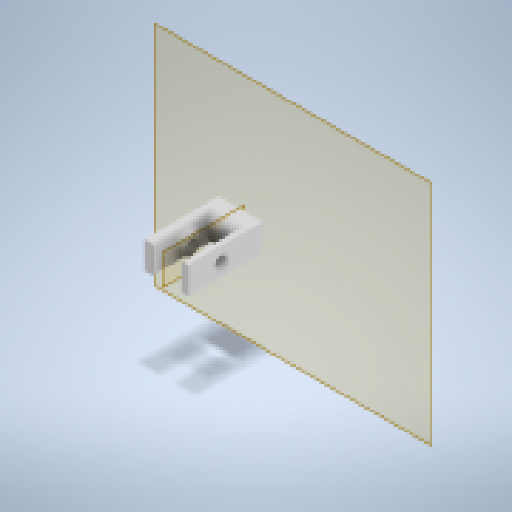
# Autodesk Inventor part: base-tensioner-head
Saved by Autodesk Inventor 2024 (Build 280153000, 153)
## iProperties
Created: 2024-03-29
Part Number: base-tensioner-head
Material: Generic
Document SubType Name: Modeling
Designer: MaartenGeorgesBuelen
Density: 1 g/cm^3
Appearance: Default
Author: MaartenGeorgesBuelen
## iProperties of the stored document base-tensioner-head_3DPrint.ipt
Created: 2024-04-17
Part Number: base-tensioner-head_3DPrint
Material: Generic
Document SubType Name: Modeling
Designer: MaartenGeorgesBuelen
Density: 1 g/cm^3
Appearance: Default
Author: MaartenGeorgesBuelen
Autodesk Inventor part; units mm, degrees
ref_plane "YZ Plane" through (0, 0, 0) normal (1, 0, 0) x (0, 1, 0)
ref_plane "XZ Plane" through (0, 0, 0) normal (0, 1, 0) x (-1, 0, 0)
ref_plane "XY Plane" through (0, 0, 0) normal (0, 0, 1) x (1, 0, 0)
ref_plane "Work Plane1" through (9.9569, 31.9885, -8.0612) normal (0, 0, 1) x (0.98136, 0.1921786, 0)
sketch "Sketch1" plane through (9.9569, 31.9885, -8.0612) normal (0, 0, 1) x (0.98136, 0.1921786, 0)
  line L0 (-81.5, 16.5) -> (-81.5, 38.5) projected
  line L1 (-53, 12.5) -> (-77.5, 12.5) projected
  line L2 (-77.5, 42.5) -> (-65, 42.5) projected
  circle A0 centre (-55.8, 18.5) radius 2.8 projected
  circle A1 centre (-72, 32.5) radius 2.1 projected
  circle A2 centre (-72, 22.5) radius 2.1 projected
  arc A3 (-77.5, 42.5) -> (-81.5, 38.5) centre (-77.5, 38.5) ccw projected
  arc A4 (-81.5, 16.5) -> (-77.5, 12.5) centre (-77.5, 16.5) ccw projected
  line L3 (-63, 2.25) -> (-63, 62.5) projected
  circle A5 centre (-55.8, 18.5) radius 3.2
  line L4 (-62.8, 13.5) -> (-48.8, 13.5)
  line L5 (-48.8, 13.5) -> (-48.8, 23.5)
  line L6 (-48.8, 23.5) -> (-62.8, 23.5)
  line L7 (-62.8, 23.5) -> (-62.8, 13.5)
  line L8 (-62.8, 13.5) -> (-48.8, 23.5) construction
  line L9 (-48.8, 13.5) -> (-62.8, 23.5) construction
  line L10 (-48.8, 23.5) -> (-46.8, 23.5)
  line L11 (-46.8, 23.5) -> (-46.8, 13.5)
  line L12 (-46.8, 13.5) -> (-48.8, 13.5)
  line L13 (-48.8, 13.5) -> (-48.8, 23.5)
  line L14 (-51, 23.5) -> (-51, 14.5) projected
  line L15 (-61, 25.5) -> (-53, 25.5) projected
  line L16 (-63, 40.5) -> (-63, 27.5) projected
  arc A6 (-63, 40.5) -> (-65, 42.5) centre (-65, 40.5) ccw projected
  arc A7 (-53, 12.5) -> (-51, 14.5) centre (-53, 14.5) ccw projected
  arc A8 (-51, 23.5) -> (-53, 25.5) centre (-53, 23.5) ccw projected
  arc A9 (-63, 27.5) -> (-61, 25.5) centre (-61, 27.5) ccw projected
  point P0 (-15.9188, -29.4787)
  dimension "d11" = 0.4
  dimension "d12" = 0.2
  dimension "d13" = 2
  dimension "d14" = 10
  constraints: 18 end point, 3 horizontal, 3 parallel, 2 midpoint, 2 perpendicular, 1 centre point, 1 collinear, 3 other
  measures "d11" radial gap between concentric circles of A0 A5
  measures "d12" distance between parallel lines of L3 L7
  measures "d13" distance of L11.end L12.end
extrude "Extrusion1" add sketch "Sketch1" along normal blind 8 contours A7 L14 L6 L5 L4 | L4 L7 L6 L14 A7 | L5 L10 L11 L12
sketch "Sketch2" plane through (9.9569, 31.9885, -0.0612) normal (0, 0, 1) x (0.98136, 0.1921786, 0)
  line L0 (-61.8, 15) -> (-49.8, 15) projected
  line L1 (-49.8, 15) -> (-49.8, 40) projected
  line L2 (-49.8, 40) -> (-61.8, 40) projected
  line L3 (-61.8, 40) -> (-61.8, 15) projected
  circle A0 centre (-55.8, 18.5) radius 3.2
  circle A1 centre (-55.8, 18.5) radius 3.2 projected
  circle A2 centre (-55.8, 18.5) radius 3.5
  point P0 (-15.9188, -29.4787)
  dimension "d21" = 0.3
  constraints: 2 centre point, 2 concentric
  measures "d21" radial gap between concentric circles of A0 A2
extrude "Extrusion2" add sketch "Sketch2" against normal blind 2 contours A2 | A0
sketch "Sketch3" plane through (9.9569, 31.9885, -0.0612) normal (0, 0, 1) x (0.98136, 0.1921786, 0)
  line L0 (-62.8, 13.5) -> (-46.8, 13.5) projected
  line L1 (-46.8, 13.5) -> (-46.8, 23.5) projected
  line L2 (-46.8, 23.5) -> (-62.8, 23.5) projected
  line L3 (-62.8, 23.5) -> (-62.8, 13.5) projected
  line L4 (-49.4, 23.5) -> (-59.4, 23.5)
  line L5 (-59.4, 23.5) -> (-59.4, 13.5)
  line L6 (-59.4, 13.5) -> (-49.4, 13.5)
  line L7 (-49.4, 13.5) -> (-49.4, 23.5)
  point P0 (-15.9188, -29.4787)
  point P1 (-49.4, 13.5)
  dimension "d15" = 10
  dimension "d16" = 2.6
  constraints: 8 end point, 2 parallel, 2 point on line, 1 horizontal, 1 perpendicular
  measures "d15" distance between parallel lines of L5 L7
  measures "d16" distance between parallel lines of L1 L7
extrude "Extrusion3" add sketch "Sketch3" along normal blind 19 contours L3 L2 L5 L0 | L7 L2 L1 L0
fillet "Fillet2" radius 4 2 edges at (-46.0234, 34.7823, -0.0612) (-47.9452, 44.5959, -0.0612)
fillet "Fillet3" radius 1 8 edges at (-41.1166, 35.7432, -2.0612) (-41.1166, 35.7432, 9.4388) (-50.9302, 33.8214, -2.0612) (-50.9302, 33.8214, 9.4388) (-52.852, 43.635, -2.0612) (-52.852, 43.635, 9.4388) (-43.0384, 45.5568, -2.0612) (-43.0384, 45.5568, 9.4388)
sketch "Sketch4" plane through (-54.2669, 33.168, -8.0612) normal (-0.98136, -0.1921786, 0) x (0, 0, 1)
  line L0 (0, 10) -> (0, 0) projected
  line L1 (0, 0) -> (27, 0) projected
  line L2 (27, 10) -> (27, 0) projected
  line L3 (0, 10) -> (27, 10) projected
  circle A0 centre (15.3, 7) radius 2.25 projected
  line L4 (27, 10) -> (25, 10)
  line L5 (25, 10) -> (25, 0)
  line L6 (25, 0) -> (27, 0)
  line L7 (27, 0) -> (27, 10)
  circle A1 centre (15.3, 5) radius 1.95
  point P0 (8.0612, -42.9787)
  dimension "d22" = 2
  dimension "d23" = 3.9
  dimension "d25" = 5
  dimension "d28" = 11.7
  constraints: 8 end point, 2 parallel, 1 centre point, 1 horizontal, 1 perpendicular, 1 point on line
  measures "d22" distance of L6.end L5.end
  measures "d23" diameter of A1
  measures "d25" distance from line of A1.centre L3
  measures "d28" distance from line of A1.centre L2
extrude "Extrusion4" cut sketch "Sketch4" against normal through all contours A1 A0 | A0 A1 picked at (15.6318, 5.4852) picked at (14.9345, 4.2325)
sketch "Sketch5" plane through (-51.699, 37.7469, -0.0612) normal (0.98136, 0.1921786, 0) x (0, 0, -1)
  circle A0 centre (-7.3, 1) radius 1.95 projected
  line L0 (8, 6) -> (8, -4) projected
  line L1 (8, -4) -> (-19, -4) projected
  line L2 (-19, 6) -> (-19, -4) projected
  line L3 (8, 6) -> (-19, 6) projected
  circle A1 centre (-7.3, 1) radius 3.45
  point P0 (-0.0612, -46.9787)
  dimension "d29" = 1.5
  constraints: 1 centre point
  measures "d29" radial gap between concentric circles of A0 A1
extrude "Extrusion5" add sketch "Sketch5" along normal blind 2 contours A1
fillet "Fillet4" radius 2.75 1 edges at (-51.8911, 38.7282, 10.6888)
ref_plane "Work Plane2" through (-46.416, 34.7054, -8.0612) normal (0.98136, 0.1921786, 0) x (0, 0, -1)
sketch "Sketch6" plane through (-41.8854, 39.6687, -0.0612) normal (-0.98136, -0.1921786, 0) x (0, 0, 1)
  circle A0 centre (7.3, 1) radius 1.95 projected
  line L0 (-8, -4) -> (-8, 6) projected
  line L1 (-8, 6) -> (19, 6) projected
  line L2 (19, -4) -> (19, 6) projected
  line L3 (-8, -4) -> (19, -4) projected
  circle A1 centre (7.3, 1) radius 3.45
  point P0 (0.0612, -46.9787)
  dimension "d33" = 1.5
  constraints: 1 centre point
  measures "d33" radial gap between concentric circles of A1 A0
extrude "Extrusion6" add sketch "Sketch6" along normal blind 2 contours A1
fillet "Fillet5" radius 2.75 1 edges at (-42.0775, 40.65, 3.7888)
move faces "Move1" translate (-2.4534, -0.4804, 0) faces at (-55.2278, 38.0748, -3.6112)
body "Solid1"
